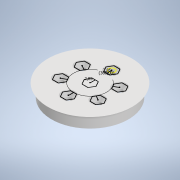
# Autodesk Inventor part: tire_cap2
Saved by Autodesk Inventor 2022 (Build 260153000, 153)
## iProperties
Created: 2023-02-08
Part Number: tire_cap2
Material: Типовые
Document SubType Name: Modeling
Designer: akapu
Density: 1 g/cm^3
Appearance: По умолчанию
Author: akapu
Autodesk Inventor part; units mm, degrees
ref_plane "YZ Plane" through (0, 0, 0) normal (1, 0, 0) x (0, 1, 0)
ref_plane "XZ Plane" through (0, 0, 0) normal (0, 1, 0) x (-1, 0, 0)
ref_plane "XY Plane" through (0, 0, 0) normal (0, 0, 1) x (1, 0, 0)
sketch "Эскиз1" plane through (0, 0, 0) normal (0, 0, 1) x (1, 0, 0)
  line L0 (-21.25, 15.93) -> (21.25, 15.93) projected
  line L1 (-16.25, 17.93) -> (-18.25, 15.93)
  line L2 (-16.25, 17.93) -> (16.25, 17.93) projected
  line L3 (16.25, 17.93) -> (18.25, 15.93)
  line L4 (-26.02, 3) -> (26.02, 3) projected
  line L5 (-21.25, 15.93) -> (-21.25, 5)
  line L6 (30, 22.93) -> (-30, 22.93) projected
  line L7 (-25.52, 22.93) -> (-25.52, 3)
  line L8 (-18.25, 15.93) -> (-18.75, 15.93)
  line L9 (0, 17.93) -> (0, 19.43)
  line L10 (-18.75, 15.93) -> (-14.5074, 15.93) construction
  line L11 (-21.25, 15.93) -> (-21.25, 22.93)
  line L12 (-21.25, 22.93) -> (0, 22.93)
  line L13 (0, 17.93) -> (0, 22.93)
  line L14 (-21.25, 15.98) -> (21.25, 15.98)
  line L15 (-18.75, 15.93) -> (-11.809, 15.93) construction
  line L16 (0, 19.43) -> (-15.25, 19.43)
  line L17 (-15.25, 19.43) -> (-18.75, 15.93)
  line L18 (-15.25, 19.43) -> (-18.75, 19.43)
  line L19 (-18.75, 19.43) -> (-18.75, 15.93)
  line L20 (21.25, 15.98) -> (21.25, 22.93)
  line L21 (0, 22.93) -> (21.25, 22.93)
  line L22 (21.75, 21.33) -> (21.75, 22.93)
  line L23 (22.25, 21.33) -> (21.25, 21.33)
  line L24 (23.25, 22.93) -> (21.25, 19.73)
  spline S0 degree 2 poles (23.25, 22.93) (21.0575, 22.6489) (21.25, 19.73) knots 0 0 0 1 1 1
  line L25 (23.25, 22.93) -> (21.25, 22.93)
  line L26 (23.25, 19.73) -> (21.25, 19.73)
  line L27 (22.25, 21.33) -> (21.25, 21.33)
  line L28 (21.75, 21.33) -> (21.75, 22.93)
  line L29 (23.25, 22.93) -> (21.25, 22.93)
  line L30 (23.25, 22.93) -> (21.25, 19.73)
  spline S1 degree 2 poles (23.25, 22.93) (21.0575, 22.6489) (21.25, 19.73) knots 0 0 0 1 1 1
  line L31 (0, 17.93) -> (-3, 17.93)
  line L32 (-3, 17.93) -> (-4.5, 19.43)
  point P0 (-18.7, 15.98)
  point P1 (-18.75, 15.98)
  point P2 (21.75, 22.13)
  point P3 (22.7031, 19.73)
  point P4 (21.75, 22.13)
  point P5 (21.25, 20.6035)
  dimension "d0" = 0.5
  dimension "d1" = 1.5
  dimension "d3" = 0.05
  dimension "d28" = 3
  constraints: 58 end point, 8 midpoint, 7 point on line, 5 perpendicular, 4 horizontal, 3 vertical, 1 collinear, 1 parallel, 14 other
  measures "d0" distance of L1.end L8.end
  measures "d1" distance of L9.start L9.end
  measures "d3" distance between parallel lines of L0 L14
  measures "d28" distance of L9.start L31.end
revolve "Вращение1" add sketch "Эскиз1" angle 360 about axis through (0, 17.93, 0) along (0, 1, 0) contours L11 L6 L13 L16 L18 L19 L14 | L16 L9 L2 L32 | L6 L22 S0 L23 L20 | L6 S0 L22 | L23 S0 L20
sketch "Эскиз3" plane through (0, 22.93, 0) normal (0, 1, 0) x (1, 0, 0)
  circle A0 centre (0, 0) radius 1.7
  line L0 (0, 0) -> (0, 12)
  circle A1 centre (0, 0) radius 21.25 projected
  circle A2 centre (0, 0) radius 15.75 projected
  circle A3 centre (0, 12) radius 1.7
  circle A4 centre (-10.3923, 6) radius 1.7
  circle A5 centre (-10.3923, -6) radius 1.7
  circle A6 centre (0, -12) radius 1.7
  circle A7 centre (10.3923, -6) radius 1.7
  circle A8 centre (10.3923, 6) radius 1.7
  point P0 (-21.25, 0)
  dimension "d7" = 3.4
  dimension "d8" = 12
  dimension "d9" = 3.4
  dimension "d12" = 360
  constraints: 7 centre point, 2 coincident, 2 end point, 1 horizontal alignment, 1 vertical, 13 other
  measures "d7" diameter of A0
  measures "d8" distance of L0.start L0.end
  measures "d9" diameter of A3
extrude "Выдавливание1" cut sketch "Эскиз3" against normal blind 10 contours A3 | A4 | A5 | A6 | A7 | A8
sketch "Эскиз4" plane through (0, 22.93, 0) normal (0, 1, 0) x (1, 0, 0)
  line L0 (0, 0) -> (0, 2.85)
  circle A0 centre (0, 12) radius 1.7 projected
  line L1 (0, 12) -> (0, 9.15)
  line L2 (1.6454, 2.85) -> (3.2909, 0)
  line L3 (3.2909, 0) -> (1.6454, -2.85)
  line L4 (1.6454, -2.85) -> (-1.6454, -2.85)
  line L5 (-1.6454, -2.85) -> (-3.2909, 0)
  line L6 (-3.2909, 0) -> (-1.6454, 2.85)
  line L7 (-1.6454, 2.85) -> (1.6454, 2.85)
  line L8 (-1.6454, 9.15) -> (-3.2909, 12)
  line L9 (-3.2909, 12) -> (-1.6454, 14.85)
  line L10 (-1.6454, 14.85) -> (1.6454, 14.85)
  line L11 (1.6454, 14.85) -> (3.2909, 12)
  line L12 (3.2909, 12) -> (1.6454, 9.15)
  line L13 (1.6454, 9.15) -> (-1.6454, 9.15)
  line L14 (8.7469, 3.15) -> (7.1014, 6)
  line L15 (10.3923, 6) -> (7.9241, 4.575)
  line L16 (12.0378, 3.15) -> (8.7469, 3.15)
  line L17 (13.6832, 6) -> (12.0378, 3.15)
  line L18 (12.0378, 8.85) -> (13.6832, 6)
  line L19 (8.7469, 8.85) -> (12.0378, 8.85)
  line L20 (7.1014, 6) -> (8.7469, 8.85)
  line L21 (7.1014, -6) -> (8.7469, -3.15)
  line L22 (10.3923, -6) -> (7.9241, -4.575)
  line L23 (8.7469, -8.85) -> (7.1014, -6)
  line L24 (12.0378, -8.85) -> (8.7469, -8.85)
  line L25 (13.6832, -6) -> (12.0378, -8.85)
  line L26 (12.0378, -3.15) -> (13.6832, -6)
  line L27 (8.7469, -3.15) -> (12.0378, -3.15)
  line L28 (-1.6454, -9.15) -> (1.6454, -9.15)
  line L29 (0, -12) -> (0, -9.15)
  line L30 (-3.2909, -12) -> (-1.6454, -9.15)
  line L31 (-1.6454, -14.85) -> (-3.2909, -12)
  line L32 (1.6454, -14.85) -> (-1.6454, -14.85)
  line L33 (3.2909, -12) -> (1.6454, -14.85)
  line L34 (1.6454, -9.15) -> (3.2909, -12)
  line L35 (-8.7469, -3.15) -> (-7.1014, -6)
  line L36 (-10.3923, -6) -> (-7.9241, -4.575)
  line L37 (-12.0378, -3.15) -> (-8.7469, -3.15)
  line L38 (-13.6832, -6) -> (-12.0378, -3.15)
  line L39 (-12.0378, -8.85) -> (-13.6832, -6)
  line L40 (-8.7469, -8.85) -> (-12.0378, -8.85)
  line L41 (-7.1014, -6) -> (-8.7469, -8.85)
  line L42 (-7.1014, 6) -> (-8.7469, 3.15)
  line L43 (-10.3923, 6) -> (-7.9241, 4.575)
  line L44 (-8.7469, 8.85) -> (-7.1014, 6)
  line L45 (-12.0378, 8.85) -> (-8.7469, 8.85)
  line L46 (-13.6832, 6) -> (-12.0378, 8.85)
  line L47 (-12.0378, 3.15) -> (-13.6832, 6)
  line L48 (-8.7469, 3.15) -> (-12.0378, 3.15)
  dimension "d16" = 2.85
  dimension "d17" = 2.85
  dimension "d20" = 360
  constraints: 98 end point, 7 coincident, 2 midpoint, 2 vertical, 123 other
  measures "d16" distance of L0.start L0.end
  measures "d17" distance of L1.start L1.end
chamfer "Фаска1" distance 2 angle 45 6 edges at (-12.0923, 22.93, -6) (-12.0923, 22.93, 6) (-1.7, 22.93, -12) (8.6923, 22.93, -6) (8.6923, 22.93, 6) (-1.7, 22.93, 12)
